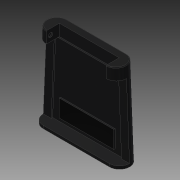
# Autodesk Inventor part: astra_clip1
Saved by Autodesk Inventor 2015 (Build 190159000, 159)
## iProperties
Created: 2016-02-10
Part Number: astra_clip1
Material: Generic
Document SubType Name: Modeling
Designer: John
Density: 1 g/cm^3
Appearance: Default
Author: John
Autodesk Inventor part; units mm, degrees
ref_plane "YZ Plane" through (0, 0, 0) normal (1, 0, 0) x (0, 1, 0)
ref_plane "XZ Plane" through (0, 0, 0) normal (0, 1, 0) x (-1, 0, 0)
ref_plane "XY Plane" through (0, 0, 0) normal (0, 0, 1) x (1, 0, 0)
sketch "Sketch3" plane through (0, 0, 0) normal (0, 1, 0) x (-1, 0, 0)
  line L0 (30, 30) -> (-30, 30)
  line L1 (-30, 30) -> (-30, -30)
  line L2 (-30, -30) -> (30, -30)
  line L3 (30, -30) -> (30, 30)
  line L4 (30, 30) -> (-30, -30) construction
  line L5 (-30, 30) -> (30, -30) construction
  line L6 (-27.5, 30) -> (27.5, 30)
  line L7 (-27.5, 30) -> (-30, -30)
  line L8 (27.5, 30) -> (30, -30)
  point P0 (0, 0)
  dimension "d7" = 60
  dimension "d8" = 60
  dimension "d9" = 2.5
  dimension "d10" = 2.5
  constraints: 19 end point, 2 midpoint, 2 parallel, 2 point on line, 1 horizontal, 1 perpendicular
  measures "d7" distance of L1.end L2.end
  measures "d8" distance of L1.end L0.end
  measures "d9" distance of L6.end L0.start
  measures "d10" distance of L0.end L6.start
extrude "Extrusion2" add sketch "Sketch3" along normal blind 14 contours L8 L2 L7 L0
fillet "Fillet1" radius 7 4 edges at (-28.75, 14, 0) (-28.75, 0, 0) (28.75, 14, 0) (28.75, 0, 0)
sketch "Sketch4" plane through (22.9939, 0, -30) normal (0, 0, -1) x (-1, 0, 0)
  ellipse E0 centre (0, 7) end of major axis (-7.0061, 7) minor radius 7 (0, 14) -> (0, 0) ccw projected
  line L0 (0, 0) -> (45.9879, 0) projected
  ellipse E1 centre (45.9879, 7) end of major axis (52.9939, 7) minor radius 7 (45.9879, 0) -> (45.9879, 14) ccw projected
  line L1 (0, 14) -> (45.9879, 14) projected
  line L2 (45.9879, 1) -> (0, 1)
  line L3 (0, 13) -> (45.9879, 13)
  spline S0 degree 5 poles (45.9879, 13) (47.0569, 13) (48.126, 12.7622) (49.1247, 12.2871) (51.2931, 10.5656) (52.2824, 7.8876) (52.2824, 6.1124) (51.2931, 3.4344) (49.1247, 1.7129) (48.126, 1.2378) (47.0569, 1) (45.9879, 1) knots 0 0 0 0 0 0 0.283434 0.283434 0.283434 0.716566 0.716566 0.716566 1 1 1 1 1 1
  spline S1 degree 5 poles (0, 1) (-1.0691, 1) (-2.1382, 1.2378) (-3.1369, 1.7129) (-5.3053, 3.4344) (-6.2945, 6.1124) (-6.2945, 7.8876) (-5.3053, 10.5656) (-3.1369, 12.2871) (-2.1382, 12.7622) (-1.0691, 13) (0, 13) knots 0 0 0 0 0 0 0.283434 0.283434 0.283434 0.716566 0.716566 0.716566 1 1 1 1 1 1
  point P0 (22.9939, 0)
  dimension "d14" = 1
  constraints: 4 end point, 3 parallel, 2 vertical alignment, 6 other
  measures "d14" distance between parallel lines of L1 L3
extrude "Extrusion3" cut sketch "Sketch4" against normal blind 0.5 contours L2 S1 L3 S0
fillet "Fillet2" radius 0.5 8 edges at (-28.9999, 7, -30) (0, 1, -30) (28.9999, 7, -30) (0, 13, -30) (-28.9999, 7, -29.5) (0, 1, -29.5) (28.9999, 7, -29.5) (0, 13, -29.5)
fillet "Fillet3" radius 0.5 4 edges at (0, 14, 30) (25.448, 11.9498, 30) (0, 0, 30) (-25.448, 11.9498, 30)
sketch "Sketch5" plane through (0, 0, 0) normal (1, 0, 0) x (0, 1, 0)
  ellipse E0 centre (7, 29.5) end of major axis (0, 29.5) minor radius 0.0208 (14, 29.5) -> (0, 29.5) ccw projected
  line L0 (14, 29.5) -> (14, -30) projected
  line L1 (14, -30) -> (0, -30) projected
  line L2 (0, -30) -> (0, 29.5) projected
  line L3 (0, -28) -> (7, -28)
  line L4 (7, -28) -> (7, 22)
  line L5 (7, 22) -> (0, 22)
  line L6 (0, 22) -> (0, -28)
  point P0 (0, 0)
  dimension "d19" = 2
  dimension "d20" = 7
  dimension "d21" = 7.5
  constraints: 8 end point, 2 parallel, 1 horizontal, 1 perpendicular, 1 point on line, 1 other
  measures "d19" distance between parallel lines of L1 L3
  measures "d20" distance of L4.end L5.end
  measures "d21" distance from line of L5 point (7, 29.5)
extrude "Extrusion4" cut sketch "Sketch5" along normal through all both and the other way through all contours L5 L4 L3 L2
sketch "Sketch7" plane through (0, 0, 0) normal (0, -1, 0) x (1, 0, 0)
  line L0 (-29.9167, -28) -> (-27.8333, 22) projected
  line L1 (-29.9167, -28) -> (29.9167, -28) projected
  line L2 (27.8333, 22) -> (29.9167, -28) projected
  line L3 (-27.8333, 22) -> (27.8333, 22) projected
  line L4 (-20.5148, 30) -> (20.5148, 30) projected
  line L5 (-20.5148, 30) -> (-20.5148, 30) projected
  line L6 (20.5148, 30) -> (-20.5148, 30) projected
  line L7 (20.5148, 30) -> (20.5148, 30) projected
  line L8 (-20.8273, 22) -> (20.8273, 22) projected
  line L9 (0, 22) -> (0, 30)
  line L10 (20.5148, 30) -> (-20.5148, 30) projected
  line L11 (-20.75, 30) -> (20.75, 30)
  line L12 (20.75, 30) -> (20.75, 22)
  line L13 (20.75, 22) -> (-20.75, 22)
  line L14 (-20.75, 22) -> (-20.75, 30)
  line L15 (-20.75, 30) -> (20.75, 22) construction
  line L16 (20.75, 30) -> (-20.75, 22) construction
  point P0 (0, 0)
  point P1 (0, 26)
  dimension "d24" = 41.5
  constraints: 14 end point, 5 midpoint, 2 parallel, 1 horizontal, 1 perpendicular, 1 point on line
  measures "d24" distance of L12.end L13.end
extrude "Extrusion5" cut sketch "Sketch7" against normal blind 9 contours L14 L11 L4 L9 L3 | L9 L4 L11 L12 L3
sketch "Sketch8" plane through (-29.9167, 7, -28) normal (0, -1, 0) x (1, 0, 0)
  line L0 (0, 0) -> (2.0833, 50) projected
  line L1 (0, 0) -> (59.8333, 0) projected
  line L2 (57.75, 50) -> (59.8333, 0) projected
  line L3 (50.6667, 50) -> (57.75, 50) projected
  line L4 (9.1667, 50) -> (50.6667, 50) projected
  line L5 (2.0833, 50) -> (9.1667, 50) projected
  line L6 (7.3589, 44.5) -> (5.7339, 5.5)
  line L7 (5.7339, 5.5) -> (54.0994, 5.5)
  line L8 (54.0994, 5.5) -> (52.4744, 44.5)
  line L9 (52.4744, 44.5) -> (50.6667, 44.5)
  line L10 (50.6667, 44.5) -> (9.1667, 44.5)
  line L11 (9.1667, 44.5) -> (7.3589, 44.5)
  line L12 (0, 0) -> (59.8333, 0) projected
  line L13 (54.3286, 0) -> (52.2452, 50)
  line L14 (9.1667, 50) -> (50.6667, 50) projected
  line L15 (29.9167, 28) -> (29.9167, 5.5)
  line L16 (5.5048, 0) -> (7.5881, 50)
  line L17 (54.3286, 0) -> (5.5048, 0)
  line L18 (50.6667, 50) -> (57.75, 50) projected
  line L19 (52.2452, 50) -> (7.5881, 50)
  dimension "d27" = 5.5
  constraints: 22 end point, 2 point on line, 2 symmetric about line, 1 collinear, 1 midpoint, 5 other
  measures "d27" distance between parallel lines of L0 L6
extrude "Extrusion6" cut sketch "Sketch8" against normal blind 1 contours L16 L7 L13 L1 | L5 L4 L3 L13 L9 L10 L11 L16 | L6 L11 L10 L9 L8 L7
sketch "Sketch9" plane through (-29.9167, 8, -28) normal (0, -1, 0) x (1, 0, 0)
  line L0 (52.2452, 50) -> (54.3286, 0) projected
  line L1 (50.6667, 50) -> (52.2452, 50) projected
  line L2 (9.1667, 50) -> (50.6667, 50) projected
  line L3 (7.5881, 50) -> (9.1667, 50) projected
  line L4 (5.5048, 0) -> (7.5881, 50) projected
  line L5 (54.3286, 0) -> (5.5048, 0) projected
  line L6 (48.9167, 3) -> (10.9167, 3)
  line L7 (10.9167, 3) -> (10.9167, 15)
  line L8 (10.9167, 15) -> (48.9167, 15)
  line L9 (48.9167, 15) -> (48.9167, 3)
  line L10 (48.9167, 3) -> (10.9167, 15) construction
  line L11 (10.9167, 3) -> (48.9167, 15) construction
  point P0 (29.9167, 28)
  point P1 (29.9167, 9)
  dimension "d30" = 38
  dimension "d31" = 12
  dimension "d32" = 3
  constraints: 12 end point, 2 midpoint, 2 parallel, 1 horizontal, 1 perpendicular
  measures "d30" distance of L7.end L8.end
  measures "d31" distance of L6.end L7.end
  measures "d32" distance between parallel lines of L6 L5
extrude "Extrusion7" add sketch "Sketch9" along normal blind 1 contours L6 L7 L8 L9
sketch "Sketch10" plane through (-20.75, 0, 23.8542) normal (1, 0, 0) x (0, 0, -1)
  ellipse E0 centre (0, 7) end of major axis (-168.1458, 7) minor radius 7 (-5.6465, 0.0039) -> (0, 0) ccw construction
  line L0 (1.8542, 0) -> (0, 0) construction
  line L1 (1.8542, 0) -> (1.8542, 8) construction
  line L2 (1.8542, 8) -> (1.8542, 9) construction
  line L3 (1.8542, 9) -> (-6.1458, 9) construction
  line L4 (-6.1458, 0.5043) -> (-6.1458, 9) construction
  line L5 (1.8542, 9) -> (-6.1458, 9) construction
  line L6 (-2.1458, 9) -> (-2.1458, 0) construction
  ellipse E1 centre (0, 7) end of major axis (-168.1458, 7) minor radius 7 (-5.6465, 0.0039) -> (0, 0) ccw construction
  line L7 (-2.1458, 9) -> (6.8542, 9) construction
  line L8 (1.8542, 4) -> (-6.1458, 4) construction
  line L9 (-6.1458, 0.5043) -> (-6.1458, 9) construction
  line L10 (-0.2854, 0) -> (-0.2854, 3) construction
  line L11 (-0.2854, 2.8772) -> (-2.1458, 2.8772) construction
  circle A0 centre (-2.1458, 2.8772) radius 1.5
  point P0 (23.8542, 0)
  point P1 (-2.1458, 4)
  dimension "d38" = 9
  dimension "d39" = 90
  dimension "d40" = 3
  dimension "d41" = 3
  constraints: 10 end point, 3 midpoint, 3 perpendicular, 3 point on line, 2 vertical, 1 centre point, 1 coincident, 1 horizontal, 5 other
  measures "d38" distance of L6.start L6.end
  measures "d39" angle of L6 L7
  measures "d40" distance of L10.start L10.end
  measures "d41" diameter of A0
extrude "Extrusion8" cut sketch "Sketch10" against normal blind 1
mirror "Mirror1" about plane through (0, 0, 0) normal (1, 0, 0) of "Extrusion8"
sketch "Sketch11" plane through (0, 14, 0) normal (0, 1, 0) x (1, 0, 0)
  line L0 (22.9939, 30) -> (-22.9939, 30) construction
  line L1 (0, 30) -> (0, 0) construction
  line L2 (12.5, 20.2686) -> (-12.5, 20.2686) construction
  line L3 (-12.5, 20.2686) -> (-12.5, 26.2686) construction
  line L4 (-12.5, 26.2686) -> (12.5, 26.2686) construction
  line L5 (12.5, 26.2686) -> (12.5, 20.2686) construction
  line L6 (12.5, 20.2686) -> (-12.5, 26.2686) construction
  line L7 (-12.5, 20.2686) -> (12.5, 26.2686) construction
  line L8 (12.5, 20.2686) -> (18.5, 20.2686)
  line L9 (18.5, 20.2686) -> (18.5, 26.2686)
  line L10 (18.5, 26.2686) -> (12.5, 26.2686)
  line L11 (12.5, 26.2686) -> (12.5, 20.2686)
  line L12 (-12.5, 20.2686) -> (-18.5, 20.2686)
  line L13 (-18.5, 20.2686) -> (-18.5, 26.2686)
  line L14 (-18.5, 26.2686) -> (-12.5, 26.2686)
  line L15 (-12.5, 26.2686) -> (-12.5, 20.2686)
  point P0 (0, 23.2686)
  dimension "d44" = 25
  dimension "d45" = 6
  dimension "d46" = 6
  dimension "d47" = 6
  dimension "d48" = 6
  dimension "d49" = 6
  constraints: 30 end point, 6 parallel, 3 horizontal, 3 midpoint, 3 perpendicular, 1 point on line, 1 vertical
  measures "d44" distance of L3.end L4.end
  measures "d45" distance of L2.end L3.end
  measures "d46" distance of L10.end L9.end
  measures "d47" distance of L9.end L8.end
  measures "d48" distance of L13.end L14.end
  measures "d49" distance of L12.end L13.end
extrude "Extrusion9" add sketch "Sketch11" along normal blind 5
fillet "Fillet4" radius 3 4 edges at (15.5, 19, -26.2686) (15.5, 19, -20.2686) (-15.5, 19, -20.2686) (-15.5, 19, -26.2686)
sketch "Sketch12" plane through (12.5, 14, -26.2686) normal (-1, 0, 0) x (0, 0, 1)
  arc A0 (6, 2) -> (0, 2) centre (3, 2) ccw projected
  line L0 (0, 0) -> (0, 2) projected
  line L1 (6, 0) -> (0, 0) projected
  line L2 (6, 0) -> (6, 2) projected
  circle A1 centre (3, 2) radius 1.5
  point P0 (26.2686, -14)
  dimension "d53" = 3
  constraints: 1 centre point, 1 coincident
  measures "d53" diameter of A1
extrude "Extrusion10" add sketch "Sketch12" along normal blind 1 contours A1
mirror "Mirror2" about plane through (0, 0, 0) normal (1, 0, 0) of "Extrusion10"
equation "\"d10\" = d9"
body "Solid2"
